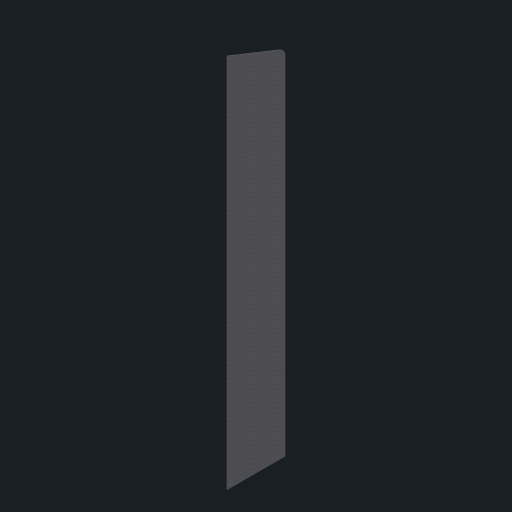
# Autodesk Inventor part: CARCASA_ALUM_2_FLAT
Saved by Autodesk Inventor 2024.3 (Build 283343000, 343)
## iProperties
Created: 2024-05-15
Part Number: CARCASA_ALUM_2_FLAT
Material: Steel, Mild, Welded
Document SubType Name: Modeling
Designer: Niler
Density: 7.85 g/cm^3
Appearance: Weld - Steel Mild
Author: Niler
Autodesk Inventor part; units mm, degrees
ref_plane "YZ Plane" through (0, 0, 0) normal (1, 0, 0) x (0, 1, 0)
ref_plane "XZ Plane" through (0, 0, 0) normal (0, 1, 0) x (-1, 0, 0)
ref_plane "XY Plane" through (0, 0, 0) normal (0, 0, 1) x (1, 0, 0)
sketch "Sketch1" plane through (0, 0, 0) normal (1, 0, 0) x (0, 1, 0)
  line L0 (1335.1265, -201.1417) -> (1415.5832, 0)
  line L1 (0, 0) -> (1415.5832, 0)
  line L2 (0, -220) -> (0, 0)
  line L3 (1307.2722, -220) -> (0, -220)
  arc A0 (1307.2722, -220) -> (1335.1265, -201.1417) centre (1307.2722, -190) ccw
  constraints: 8 end point, 2 horizontal, 2 point on circle, 1 centre point, 1 coincident, 1 vertical, 9 other
extrude "Extrusion1" add sketch "Sketch1" along normal blind 1.5
body "Solid1"
